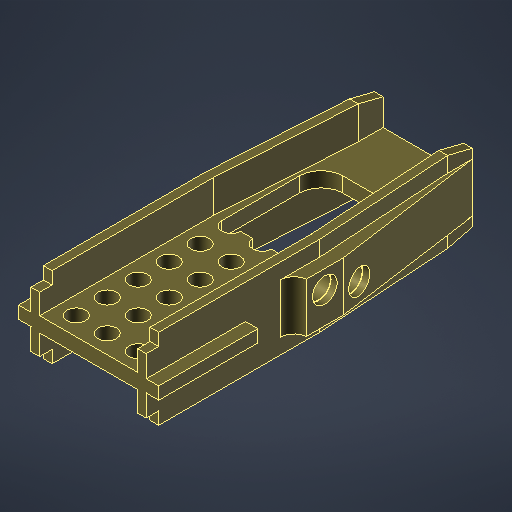
# Autodesk Inventor part: Payload_NP1
Saved by Autodesk Inventor 2026.2 (Build 302298000, 298)
## iProperties
Created: 2021-05-04
Part Number: Payload_NP1
Material: Nylon 6/6
Document SubType Name: Modeling
Designer: Pip
Density: 1.13 g/cm^3
Appearance: Nylon 6
Mass: 0.385973 g
Surface Area: 10.1509 cm^2
Volume: 0.341569 cm^3
WallThickness: 0.700 mm
InterProbeDist: 2.500 mm
Author: Pip
Autodesk Inventor part; units mm, degrees
ref_plane "YZ Plane" through (0, 0, 0) normal (1, 0, 0) x (0, 1, 0)
ref_plane "XZ Plane" through (0, 0, 0) normal (0, 1, 0) x (-1, 0, 0)
ref_plane "XY Plane" through (0, 0, 0) normal (0, 0, 1) x (1, 0, 0)
sketch "Sk:Base" plane through (0, 0, 0) normal (0, 1, 0) x (-1, 0, 0)
  line L0 (0, -7) -> (-3.95, -7)
  line L1 (-3.95, -7) -> (-3.95, 7)
  line L2 (-3.95, 7) -> (0, 7)
  line L3 (0, 7) -> (0, -7)
  line L4 (-3.95, -7) -> (-3.25, -18)
  line L5 (-3.25, -18) -> (0, -18)
  line L6 (0, -18) -> (0, -7)
  line L7 (-3.95, 7) -> (-4.65, 7)
  line L8 (-4.65, -7) -> (-3.95, -7)
  line L9 (-3.95, -7) -> (-3.95, 7)
  line L10 (-3.95, -18) -> (-3.25, -18)
  line L11 (0, 7) -> (-2.5, 7)
  line L12 (-4.65, -7) -> (-4.65, 7)
  line L13 (-4.65, -7) -> (-3.95, -18)
  line L14 (-3.25, -18) -> (-3.25, -7)
  line L15 (-5.65, -4.9039) -> (-4.65, -4.9039)
  line L16 (-5.65, -4.9039) -> (-5.65, -7.9039)
  line L17 (-4.65, 7) -> (-5.65, 7)
  line L18 (-5.65, 7) -> (-5.65, -1)
  line L19 (-5.65, -1) -> (-4.65, -1)
  line L20 (-4.65, -1) -> (-4.65, 7)
  line L21 (-3.95, -18) -> (-3.25, -18)
  line L22 (-3.25, -18) -> (-3.25, -20)
  line L23 (-3.25, -20) -> (-3.95, -20)
  line L24 (-3.95, -20) -> (-3.95, -18)
  line L25 (-3.25, -20) -> (0, -20)
  line L26 (0, -20) -> (0, -15)
  line L27 (-3.25, -18.5) -> (-3.25, -20)
  line L28 (-3.95, -20) -> (-5.65, -7.9039)
  line L29 (0, -15) -> (-3.4409, -15)
  point P0 (0, 0)
  point P1 (-4.65, -1)
  point P2 (0, -15)
  point P3 (-3.25, -15)
  dimension "d0" = 3.95
  dimension "d11" = 14
  dimension "d2" = 0
  dimension "d6" = 3.25
  dimension "d7" = 0
  dimension "d1" = 0.7
  dimension "d40" = 7
  dimension "d41" = 11
  dimension "d129" = 3
  dimension "d148" = 8
  dimension "d167" = 2
  dimension "d168" = 0.7
  dimension "d172" = 1
  dimension "d173" = 1
  dimension "d194" = 0
  dimension "d233" = 5
  dimension "d234" = 8
  constraints: 60 end point, 9 parallel, 8 horizontal, 6 perpendicular, 4 point on line, 3 vertical
  measures "d0" distance of L0.start L0.end
  measures "d11" distance of L0.end L1.end
  measures "d2" distance from line of point (0, 0) L3
  measures "d6" distance of L4.end L5.end
  measures "d7" horizontal distance of L0.start L5.end
  measures "d1" distance between parallel lines of L12 L1
  measures "d40" distance from line of point (0, 0) L2
  measures "d41" distance between parallel lines of L0 L5
  measures "d129" distance of L15.start L16.end
  measures "d148" distance of L17.end L18.end
  measures "d167" distance of L21.end L22.end
  measures "d168" distance between parallel lines of L24 L22
  measures "d172" distance between parallel lines of L12 L18
  measures "d173" distance between parallel lines of L12 L16
  measures "d194" distance from line of point (0, 0) L26
  measures "d233" distance of L25.end L26.end
  measures "d234" angle of L14 L28
extrude "Ex:Midline" add sketch "Sk:Base" along normal blind 0.6 contours L0 L1 L2 L3 | L14 L29 L4 L0 | L14 L4 L29
extrude "Ex:FrontSupport" add sketch "Sk:Base" along normal blind 0.6 contours L6 L5 L14 L29 | L26 L25 L22 L5
extrude "Ex:SideRidge" add sketch "Sk:Base" along normal blind 0.5 contours L12 L19 L18 L17
extrude "Ex:SideWall" add sketch "Sk:Base" along normal blind 3.25 contours L8 L12 L7 L1 | L4 L10 L13 L8 | L22 L23 L24 L10
sketch "Sketch12" plane through (0, 0.6, 0) normal (0, 1, 0) x (1, 0, 0)
  circle A0 centre (2.5, -5.5) radius 0.75
  line L0 (0, -7) -> (3.95, -7) projected
  line L1 (0, 7) -> (0, -7) projected
  point P0 (0, 0)
  point P1 (0, 10)
  dimension "d68" = 1.5
  dimension "d69" = 1.5
  dimension "d79" = 2.5
  constraints: 1 centre point
  measures "d68" diameter of A0
  measures "d69" distance from line of A0.centre L0
  measures "d79" distance from line of A0.centre L1
extrude "Ex:BaseHole" cut sketch "Sketch12" against normal mid plane 5.3
pattern_linear "Pat:BaseHoles" count 6 spacing 2.5 along (0, 0, -1) count 3 spacing 2.5 along (-1, 0, 0) of "Ex:BaseHole"
fillet "Fillet:Support" radius 1.75 1 edges at (3.25, 0.3, -15)
extrude "Ex:Widening" add sketch "Sk:Base" along normal blind 2 contours L13 L24 L28 L16 L15 L12 | L22 L23 L24 L10
fillet "Fillet:Side" radius 1.1 1 edges at (4.65, 1, -4.9039)
sketch "Sketch24" plane through (3.95, 3.25, -18) normal (1, 0, 0) x (0, 0, -1)
  line L0 (2, 0) -> (0, 0) projected
  line L1 (0, -1.25) -> (2, -1.25) projected
  line L2 (0, 0) -> (2, 0)
  line L3 (2, 0) -> (2, -1.25)
  line L4 (2, -1.25) -> (0, -1.25)
  line L5 (0, -1.25) -> (0, 0)
  line L6 (0, 0) -> (-11, 0) projected
  line L7 (0, 0) -> (2, -0.5)
  point P0 (-18, -3.25)
  point P1 (5.5, 0)
  point P2 (4.5, 0)
  dimension "d219" = 1.25
  dimension "d222" = 0.5
  dimension "d223" = 0
  constraints: 10 end point, 2 parallel, 1 horizontal, 1 perpendicular
  measures "d219" distance of L4.end L0.end
  measures "d222" distance of L0.start L7.end
  measures "d223" distance from line of L3 L7.end
extrude "Ex:FrontTaper" cut sketch "Sketch24" against normal up to next contours L3 L7 L0
sketch "Sk:LidNotch" plane through (4.65, 0.5, 7) normal (1, 0, 0) x (0, 0, -1)
  line L0 (0, 0.1) -> (0, 2.75) projected
  line L1 (0, 2.75) -> (1, 2.75)
  line L2 (1, 2.75) -> (1, 1.75)
  line L3 (1, 1.75) -> (0, 1.75)
  line L4 (0, 1.75) -> (0, 2.75)
  line L5 (0, 2.75) -> (14, 2.75) projected
  point P0 (7, -0.5)
  point P1 (0, 1.75)
  dimension "d224" = 1
  dimension "d225" = 1
  constraints: 8 end point, 2 parallel, 1 horizontal, 1 perpendicular
  measures "d224" distance between parallel lines of L0 L2
  measures "d225" distance between parallel lines of L5 L3
extrude "Ex:LidNotch" cut sketch "Sk:LidNotch" against normal up to next
mirror "Mirror1" about plane through (0, 0, -7) normal (-1, 0, 0)
mirror "Mirror2" about plane through (1.975, 0, 0) normal (0, -1, 0)
sketch "Sk:ThreadHole1" plane through (5.65, 2, -4.9039) normal (1, 0, 0) x (0, 0, -1)
  circle A0 centre (1.5, -1.5) radius 0.95
  circle A1 centre (1.5, -1.5) radius 1
  line L0 (0, 0) -> (3, 0) projected
  line L1 (0, -4) -> (0, 0) projected
  point P0 (-4.9039, -2)
  point P1 (0, -2)
  point P2 (0, -1.5)
  dimension "d130" = 1.9
  dimension "d131" = 2
  dimension "d199" = 1.5
  dimension "d200" = 1.5
  constraints: 2 centre point, 1 concentric
  measures "d130" diameter of A0
  measures "d131" diameter of A1
  measures "d199" distance from line of L0 A0.centre
  measures "d200" distance from line of L1 A0.centre
sketch "Sk:ThreadHole2" plane through (4.7435, -2, -14.3541) normal (0.9902681, 0, -0.1391731) x (-0.1391731, 0, -0.9902681)
  circle A0 centre (-5.0136, 1.5) radius 1
  circle A1 centre (-5.0136, 1.5) radius 0.95
  line L0 (-6.5136, 0) -> (5.7014, 0) projected
  line L1 (-6.5136, 0) -> (-6.5136, 4) projected
  point P0 (-13.5543, 2)
  dimension "d134" = 1.9
  dimension "d135" = 2
  dimension "d217" = 1.5
  dimension "d232" = 1.5
  constraints: 2 centre point, 1 concentric
  measures "d134" diameter of A1
  measures "d135" diameter of A0
  measures "d217" distance from line of L0 A0.centre
  measures "d232" distance from line of L1 A0.centre
extrude "Ex:ThreadHole1" cut sketch "Sk:ThreadHole1" against normal blind 1.5 contours A0
extrude "Ex:ThreadEntry1" cut sketch "Sk:ThreadHole1" against normal blind 0.5 contours A0 | A1
extrude "Ex:ThreadHole2" cut sketch "Sk:ThreadHole2" against normal blind 1.5 contours A1
extrude "Ex:ThreadEntry2" cut sketch "Sk:ThreadHole2" against normal blind 0.5 contours A0 | A1
pattern_circular "Pat:Threads" count 2 over 360 about axis through (0, 0, -10) along (0, 0, 1) of "Ex:ThreadEntry1", "Ex:ThreadEntry2", "Ex:ThreadHole2", "Ex:ThreadHole1"
equation "\"d40\" = 0.5 * d11"
equation "\"SideWallHeight\" = 3.25"
body "Solid1"
